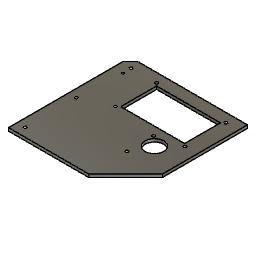
ECE198 Housing v1-7 (Autodesk Fusion 360 archive; units mm, degrees)
design "Lid"
Autodesk Fusion 360 part; units mm, degrees
note: some values were not read from the file. Set by a fixed rule: the direction of a hole.
other "DerivedContext1"
sketch "lid v2" plane through (-180, 0, 0) normal (0, 0, 1) x (1, 0, 0)
  line L0 (334.0338, -3.2613) -> (192.2917, -3.2613)
  line L1 (316.9875, -15.8281) -> (316.9875, -64.0063)
  line L2 (287.0338, -159.4636) -> (334.0338, -112.4636)
  line L3 (231.1593, -15.8281) -> (316.9875, -15.8281)
  line L4 (337.6529, -114.5635) -> (288.1529, -164.0635)
  line L5 (192.2917, -3.2613) -> (183.2917, -12.2613)
  line L6 (334.0338, -112.4636) -> (334.0338, -3.2613)
  line L7 (183.2917, -12.2613) -> (183.2917, -159.4636)
  line L8 (316.9875, -64.0063) -> (231.1593, -64.0063)
  line L9 (183.2917, -159.4636) -> (287.0338, -159.4636)
  line L10 (180, -164.0635) -> (180, -10.5)
  line L11 (288.1529, -164.0635) -> (180, -164.0635)
  line L12 (180, -10.5) -> (190.5, 0)
  line L13 (337.6529, 0) -> (337.6529, -114.5635)
  line L14 (190.5, 0) -> (337.6529, 0)
  circle A0 centre (299.8198, -87.3938) radius 12.5
  line L15 (231.1593, -64.0063) -> (231.1593, -15.8281)
extrude "Extrude3" add sketch "lid v2" along normal blind 4 contours L0 L2 L5 L6 L7 L9 | L4 L10 L11 L12 L13 L14
sketch "holes" plane through (0, 0, 0) normal (0, 0, 1) x (1, 0, 0)
  circle A0 centre (107.319, -111.8847) radius 1.8365
  circle A1 centre (47.5029, -67.3964) radius 1.8365
  circle A2 centre (32.3241, -70.8602) radius 1.0037
  circle A3 centre (140.7271, -67.3151) radius 1.8365
  circle A4 centre (32.3241, -31.7681) radius 1.0037
  circle A5 centre (10.805, -83.5722) radius 1.8365
  circle A6 centre (32.3241, -70.8602) radius 1.0037
  circle A7 centre (47.5029, -67.3964) radius 1.8365
  circle A8 centre (13.6288, -23.4202) radius 1.4371
  circle A9 centre (10.8512, -152.3487) radius 1.8365
  circle A10 centre (140.7255, -12.2643) radius 1.8365
  circle A11 centre (47.5569, -12.2533) radius 1.8365
  circle A12 centre (11.9504, -31.7681) radius 1.0037
  circle A13 centre (47.5029, -67.3964) radius 1.8365
  circle A14 centre (13.2779, -12.3099) radius 1.8365
  circle A15 centre (107.3816, -76.1037) radius 1.8365
  circle A16 centre (11.9504, -70.8602) radius 1.0037
  circle A17 centre (47.5029, -67.3964) radius 1.8365
hole "Hole1" at (13.2779, -12.3099, 0) at (47.5029, -67.3964, 0) at (10.8512, -152.3487, 0) at (107.319, -111.8847, 0) at (107.3816, -76.1037, 0) at (140.7271, -67.3151, 0) at (140.7255, -12.2643, 0) at (10.805, -83.5722, 0) at (47.5569, -12.2533, 0) direction (0, 0, 1) diameter 3.783 depth 15 tip angle 180
thread "Thread1" "ISO Metric profile 4.5 M4.5x0.75 6H"
hole "Hole2" at (13.6288, -23.4202, 0) direction (0, 0, 1) diameter 3 depth 8 tip angle 180
